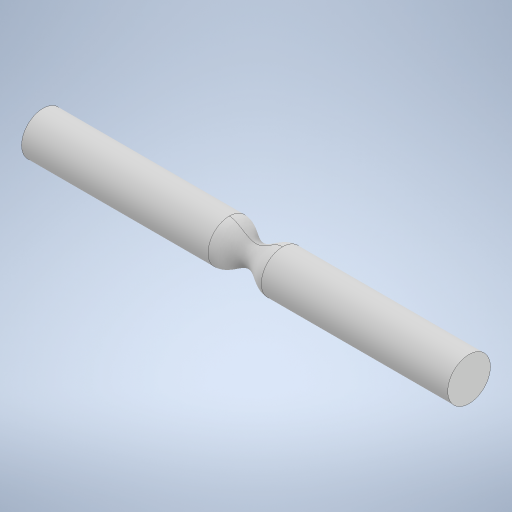
# Autodesk Inventor part: stenosis_1
Saved by Autodesk Inventor 2024 (Build 280153000, 153)
## iProperties
Created: 2023-05-05
Part Number: stenosis_1
Material: Generic
Document SubType Name: Modeling
Designer: csala
Density: 1 g/cm^3
Appearance: Default
Author: csala
Autodesk Inventor part; units mm, degrees
ref_plane "YZ Plane" through (0, 0, 0) normal (1, 0, 0) x (0, 1, 0)
ref_plane "XZ Plane" through (0, 0, 0) normal (0, 1, 0) x (-1, 0, 0)
ref_plane "XY Plane" through (0, 0, 0) normal (0, 0, 1) x (1, 0, 0)
sketch "Sketch1" plane through (0, 0, 0) normal (0, 0, 1) x (1, 0, 0)
  line L0 (0, 0) -> (40, 0)
  line L1 (40, 0) -> (40, 2)
  line L2 (0, 0) -> (0, 2)
  line L3 (0, 2) -> (17.5, 2)
  spline S0 degree 5 poles (17.5, 2) (17.7732, 2.0015) (18.0468, 1.9206) (18.2872, 1.7904) (18.7501, 1.4994) (19.2126, 1.2106) (19.4535, 1.0776) (20, 0.9218) (20.5465, 1.0776) (20.7874, 1.2106) (21.2499, 1.4994) (21.7128, 1.7904) (21.9532, 1.9206) (22.2268, 2.0015) (22.5, 2) knots 0 0 0 0 0 0 0.25 0.25 0.25 0.5 0.5 0.5 0.75 0.75 0.75 1 1 1 1 1 1
  line L4 (40, 2) -> (22.5, 2)
  dimension "L" = 40
  dimension "r" = 2
  constraints: 10 end point, 2 equal length, 2 horizontal, 2 perpendicular, 1 collinear, 4 other
  measures "L" distance of L0.start L0.end
  measures "r" distance of L0.start L2.end
revolve "Revolution1" add sketch "Sketch1" angle 360 about axis through (0, 0, 0) along (1, 0, 0)
equation "\"r_min\" = 1"
equation "\"L_st\" = 5"
equation "curve S0 of \"Sketch1\": x = t; y = r_min + (r - r_min)*sin(180*t/L_st*1mm)^2; t from d2 to d3"
body "Solid1"
